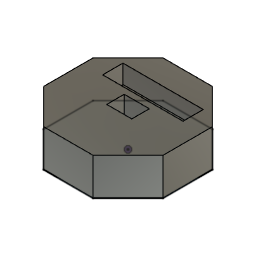
TimeSphereV1 (Autodesk Fusion 360 design; units mm, degrees)
Autodesk Fusion 360 part; units mm, degrees
sketch "Sketch1" plane through (0, 0, 0) normal (0, 0, 1) x (1, 0, 0)
  line L0 (61.321, 25.4) -> (25.4, 61.321)
  line L1 (25.4, 61.321) -> (-25.4, 61.321)
  line L2 (-25.4, 61.321) -> (-61.321, 25.4)
  line L3 (-61.321, 25.4) -> (-61.321, -25.4)
  line L4 (-61.321, -25.4) -> (-25.4, -61.321)
  line L5 (-25.4, -61.321) -> (25.4, -61.321)
  line L6 (25.4, -61.321) -> (61.321, -25.4)
  line L7 (61.321, -25.4) -> (61.321, 25.4)
  dimension "d1" = 50.8
  constraint horizontal L1
  measures "d1" distance of L4.end L5.end
extrude "Extrude1" add sketch "Sketch1" along normal blind 38.1
sketch "Sketch6" plane through (0, 0, 38.1) normal (0, 0, 1) x (-1, 0, 0)
  line L0 (-61.321, 25.4) -> (-61.321, -25.4)
  line L1 (-61.321, -25.4) -> (-25.4, -61.321)
  line L2 (-25.4, -61.321) -> (25.4, -61.321)
  line L3 (25.4, -61.321) -> (61.321, -25.4)
  line L4 (61.321, -25.4) -> (61.321, 25.4)
  line L5 (61.321, 25.4) -> (25.4, 61.321)
  line L6 (25.4, 61.321) -> (-25.4, 61.321)
  line L7 (-25.4, 61.321) -> (-61.321, 25.4)
  line L8 (-12.8905, 9.017) -> (12.8905, 9.017)
  line L9 (12.8905, 9.017) -> (12.8905, -9.017)
  line L10 (12.8905, -9.017) -> (-12.8905, -9.017)
  line L11 (-12.8905, -9.017) -> (-12.8905, 9.017)
  line L12 (-12.8905, 9.017) -> (12.8905, -9.017) construction
  line L13 (12.8905, 9.017) -> (-12.8905, -9.017) construction
  dimension "d28" = 25.781
  dimension "d29" = 18.034
  constraint horizontal L8
  constraint perpendicular L8 L9
  constraint parallel L8 L10
  constraint parallel L9 L11
  constraint coincident L12 origin
  constraint coincident L13 origin
  measures "d28" distance of L9.end L10.end
  measures "d29" distance of L8.end L9.end
extrude "Extrude12" cut sketch "Sketch6" against normal blind 19.05 contours L8 L9 L10 L11
sketch "Sketch7" plane through (0, 0, 19.05) normal (0, 0, 1) x (-1, 0, 0)
  line L0 (-12.8905, -9.017) -> (12.8905, -9.017)
  line L1 (12.8905, -9.017) -> (12.8905, 9.017)
  line L2 (12.8905, 9.017) -> (-12.8905, 9.017)
  line L3 (-12.8905, 9.017) -> (-12.8905, -9.017)
  circle A0 centre (10.16, -6.35) radius 0.85
  dimension "d40" = 1.7
  dimension "d41" = 10.16
  dimension "d42" = 6.35
  measures "d40" diameter of A0
  measures "d41" horizontal distance of origin A0.centre
  measures "d42" vertical distance of origin A0.centre
extrude "Extrude13" cut sketch "Sketch7" against normal blind 6.35 contours A0
sketch "Sketch8" plane through (0, 0, 19.05) normal (0, 0, 1) x (-1, 0, 0)
  circle A0 centre (10.16, -6.35) radius 0.85
  line L0 (-12.8905, -9.017) -> (12.8905, -9.017)
  line L1 (12.8905, -9.017) -> (12.8905, 9.017)
  line L2 (12.8905, 9.017) -> (-12.8905, 9.017)
  line L3 (-12.8905, 9.017) -> (-12.8905, -9.017)
  line L4 (0, -11.43) -> (0, 10.8522)
  line L5 (13.97, 0) -> (-13.97, 0)
  circle A1 centre (-10.16, -6.35) radius 0.85
  circle A2 centre (10.16, 6.35) radius 0.85
  circle A3 centre (-10.16, 6.35) radius 0.85
  constraint perpendicular L2 L4
  constraint perpendicular L3 L5
  constraint symmetric A0 L4 A1
  constraint symmetric A0 L5 A2
  constraint symmetric L5 A1 A3
extrude "Extrude14" cut sketch "Sketch8" against normal blind 6.35 contours A1 | A2 | A3
sketch "Sketch9" plane through (0, 0, 19.05) normal (0, 0, 1) x (-1, 0, 0)
  circle A0 centre (-10.16, -6.35) radius 0.85
  circle A1 centre (-10.16, 6.35) radius 0.85
  circle A2 centre (10.16, 6.35) radius 0.85
  circle A3 centre (10.16, -6.35) radius 0.85
  line L0 (-12.8905, -9.017) -> (12.8905, -9.017)
  line L1 (12.8905, -9.017) -> (12.8905, 9.017)
  line L2 (12.8905, 9.017) -> (-12.8905, 9.017)
  line L3 (-12.8905, 9.017) -> (-12.8905, -9.017)
  line L4 (7.874, 5.0932) -> (-7.874, 5.0932)
  line L5 (-7.874, 5.0932) -> (-7.874, 8.2682)
  line L6 (-7.874, 8.2682) -> (7.874, 8.2682)
  line L7 (7.874, 8.2682) -> (7.874, 5.0932)
  dimension "d45" = 15.748
  dimension "d46" = 3.175
  dimension "d47" = 7.874
  constraint horizontal L4
  constraint vertical L5
  constraint horizontal L6
  constraint vertical L7
  measures "d45" distance of L4.start L4.end
  measures "d46" distance of L4.end L5.end
  measures "d47" distance of origin L5
extrude "Extrude15" cut sketch "Sketch9" against normal blind 5.08 contours L4 L5 L6 L7
sketch "Sketch10" plane through (0, 0, 38.1) normal (0, 0, 1) x (-1, 0, 0)
  line L0 (12.8905, 9.017) -> (12.8905, -9.017)
  line L1 (12.8905, -9.017) -> (-12.8905, -9.017)
  line L2 (-12.8905, -9.017) -> (-12.8905, 9.017)
  line L3 (-12.8905, 9.017) -> (12.8905, 9.017)
  line L4 (-61.321, 25.4) -> (-61.321, -25.4)
  line L5 (-61.321, -25.4) -> (-25.4, -61.321)
  line L6 (-25.4, -61.321) -> (25.4, -61.321)
  line L7 (25.4, -61.321) -> (61.321, -25.4)
  line L8 (61.321, -25.4) -> (61.321, 25.4)
  line L9 (61.321, 25.4) -> (25.4, 61.321)
  line L10 (25.4, 61.321) -> (-25.4, 61.321)
  line L11 (-25.4, 61.321) -> (-61.321, 25.4)
  line L12 (41.275, -36.068) -> (-41.275, -36.068)
  line L13 (-41.275, -36.068) -> (-41.275, -15.24)
  line L14 (-41.275, -15.24) -> (41.275, -15.24)
  line L15 (41.275, -15.24) -> (41.275, -36.068)
  line L16 (41.275, -36.068) -> (-41.275, -15.24) construction
  line L17 (-41.275, -36.068) -> (41.275, -15.24) construction
  point P0 (0, -25.654)
  dimension "d50" = 82.55
  dimension "d51" = 20.828
  dimension "d52" = 15.24
  constraint horizontal L12
  constraint perpendicular L12 L13
  constraint parallel L12 L14
  constraint parallel L13 L15
  constraint coincident L16 P0
  constraint coincident L17 P0
  constraint vertical origin P0
  measures "d50" distance of L12.start L12.end
  measures "d51" distance of L12.start L14.end
  measures "d52" distance of origin L14
extrude "Extrude16" cut sketch "Sketch10" against normal blind 19.05 contours L12 L13 L14 L15
equation "d47 = ( 0.62 / 2 ) * 1 in"
